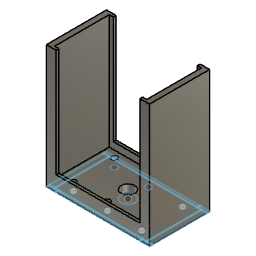
KaiserStandBracket v10 (Autodesk Fusion 360 design; units mm, degrees)
Autodesk Fusion 360 part; units mm, degrees
sketch "Schizzo1" plane through (0, 0, 0) normal (0, 0, 1) x (1, 0, 0)
  line L0 (20.7879, 45.3781) -> (88.2879, 45.3781)
  line L1 (88.2879, 45.3781) -> (88.2879, 5.3781)
  line L2 (88.2879, 5.3781) -> (20.7879, 5.3781)
  line L3 (20.7879, 5.3781) -> (20.7879, 45.3781)
  line L4 (20.7879, 45.3781) -> (16.7879, 45.3781)
  line L5 (16.7879, 45.3781) -> (16.7879, 5.3781)
  line L6 (16.7879, 5.3781) -> (20.7879, 5.3781)
  line L7 (20.7879, 5.3781) -> (20.7879, 45.3781)
  line L8 (54.5379, 45.3781) -> (54.5379, 5.3781) construction
  line L9 (88.2879, 25.3781) -> (20.7879, 25.3781) construction
  line L10 (92.2879, 45.3781) -> (92.2879, 5.3781)
  line L11 (88.2879, 5.3781) -> (88.2879, 45.3781)
  line L12 (92.2879, 5.3781) -> (88.2879, 5.3781)
  line L13 (88.2879, 45.3781) -> (92.2879, 45.3781)
  line L14 (79.5379, 10.3781) -> (29.5379, 10.3781) construction
  line L15 (29.5379, 10.3781) -> (29.5379, 40.3781) construction
  line L16 (29.5379, 40.3781) -> (79.5379, 40.3781) construction
  line L17 (79.5379, 40.3781) -> (79.5379, 10.3781) construction
  line L18 (79.5379, 10.3781) -> (29.5379, 40.3781) construction
  line L19 (29.5379, 10.3781) -> (79.5379, 40.3781) construction
  circle A0 centre (29.5379, 40.3781) radius 2.05
  circle A1 centre (79.5379, 40.3781) radius 2.05
  circle A2 centre (29.5379, 10.3781) radius 2.05
  circle A3 centre (79.5379, 10.3781) radius 2.05
  circle A4 centre (54.5379, 40.3781) radius 2.05
  circle A5 centre (54.5379, 10.3781) radius 2.05
  line L20 (16.7879, 5.3781) -> (23.7879, 5.3781)
  line L21 (23.7879, 5.3781) -> (23.7879, 3.3781)
  line L22 (23.7879, 3.3781) -> (16.7879, 3.3781)
  line L23 (16.7879, 3.3781) -> (16.7879, 5.3781)
  line L24 (16.7879, 45.3781) -> (23.7879, 45.3781)
  line L25 (23.7879, 47.3781) -> (16.7879, 47.3781)
  line L26 (23.7879, 45.3781) -> (23.7879, 47.3781)
  line L27 (16.7879, 47.3781) -> (16.7879, 45.3781)
  line L28 (92.2879, 45.3781) -> (85.2879, 45.3781)
  line L29 (92.2879, 5.3781) -> (85.2879, 5.3781)
  line L30 (85.2879, 3.3781) -> (92.2879, 3.3781)
  line L31 (85.2879, 5.3781) -> (85.2879, 3.3781)
  line L32 (92.2879, 3.3781) -> (92.2879, 5.3781)
  line L33 (85.2879, 47.3781) -> (92.2879, 47.3781)
  line L34 (85.2879, 45.3781) -> (85.2879, 47.3781)
  line L35 (92.2879, 47.3781) -> (92.2879, 45.3781)
  circle A6 centre (54.5379, 25.3781) radius 5
  line L36 (23.7879, 5.3781) -> (85.2879, 5.3781)
  line L37 (85.2879, 5.3781) -> (85.2879, 3.3781)
  line L38 (85.2879, 3.3781) -> (23.7879, 3.3781)
  line L39 (23.7879, 3.3781) -> (23.7879, 5.3781)
  line L40 (23.7879, 47.3781) -> (85.2879, 47.3781)
  line L41 (85.2879, 47.3781) -> (85.2879, 45.3781)
  line L42 (85.2879, 45.3781) -> (23.7879, 45.3781)
  line L43 (23.7879, 45.3781) -> (23.7879, 47.3781)
  point P0 (54.5379, 25.3781)
  dimension "d1" = 67.5
  dimension "d2" = 40
  dimension "d3" = 4
  dimension "d4" = 50
  dimension "d5" = 30
  dimension "d6" = 4.1
  dimension "d8" = 4.1
  dimension "d13" = 7
  dimension "d14" = 2
  dimension "d15" = 10
  dimension "d19" = 7
  dimension "d20" = 75.5
  constraint horizontal L0
  constraint vertical L1
  constraint horizontal L2
  constraint vertical L3
  constraint horizontal L4
  constraint vertical L5
  constraint horizontal L6
  constraint vertical L7
  constraint coincident L2.end L3.start
  constraint midpoint L0 L8.start
  constraint midpoint L2 L8.end
  constraint midpoint L1 L9.start
  constraint midpoint L7 L9.end
  constraint symmetric L0.start L8 L0.end
  constraint symmetric L4.end L8 L10.start
  constraint symmetric L5.end L8 L10.end
  constraint symmetric L2.end L8 L1.end
  constraint horizontal L14
  constraint perpendicular L14 L15
  constraint parallel L14 L16
  constraint parallel L15 L17
  constraint coincident L18 P0
  constraint coincident L19 P0
  constraint midpoint L8 P0
  constraint coincident L15.end L16.start
  constraint symmetric L8 A0 A1
  constraint symmetric L9 A0 A2
  constraint symmetric L9 A1 A3
  constraint midpoint L16 A4.centre
  constraint symmetric L9 A4 A5
  constraint horizontal L20
  constraint vertical L21
  constraint horizontal L22
  constraint vertical L23
  constraint symmetric L5.end L9 L4.end
  constraint symmetric L9 L20.end L24.end
  constraint symmetric L9 L21.end L25.start
  constraint symmetric L9 L22.end L25.end
  constraint symmetric L8 L20.end L29.end
  constraint symmetric L8 L21.end L30.start
  constraint symmetric L8 L22.end L30.end
  constraint symmetric L8 L4.end L10.start
  constraint symmetric L8 L24.end L28.end
  constraint symmetric L8 L25.start L33.start
  constraint symmetric L8 L25.end L33.end
  constraint coincident P0 A6.centre
  constraint horizontal L36
  constraint vertical L37
  constraint horizontal L38
  constraint vertical L39
  constraint coincident L30.start L31.end
  constraint horizontal L40
  constraint vertical L41
  constraint horizontal L42
  constraint vertical L43
  constraint coincident L28.end L34.start
  measures "d1" distance of L0.start L0.end
  measures "d2" distance of L0.start L2.end
  measures "d3" distance of L0.start L4.end
  measures "d4" distance of L15.end L16.end
  measures "d5" distance of L14.end L15.end
  measures "d6" diameter of A0
  measures "d8" diameter of A4
  measures "d13" distance of L5.end L20.end
  measures "d14" distance of L5.end L22.end
  measures "d15" diameter of A6
  measures "d19" distance of L14.start L38
  measures "d20" distance of L5 L10
extrude "Estrusione1" add sketch "Schizzo1" along normal blind 6 contours L0 L1 L2 L3 L7 L11 L20 L24 L28 L29 L36 L42 | L0 L26 L34 L40 L41 L42 L43 | L2 L21 L31 L36 L37 L38 L39
extrude "Estrusione2" add sketch "Schizzo1" along normal blind 90 contours L0 L4 L24 L25 L26 L27 L43 | L3 L4 L5 L6 L7 L20 L24 | L2 L6 L20 L21 L22 L23 L39 | L0 L13 L28 L33 L34 L35 L41 | L1 L10 L11 L12 L13 L28 L29 | L2 L12 L29 L30 L31 L32 L37
extrude "Estrusione3" add sketch "Schizzo1" along normal blind 5 from surface at 6 contours L0 L26 L34 L40 L41 L42 L43 | L2 L21 L31 L36 L37 L38 L39
equation "d8 = d6"
